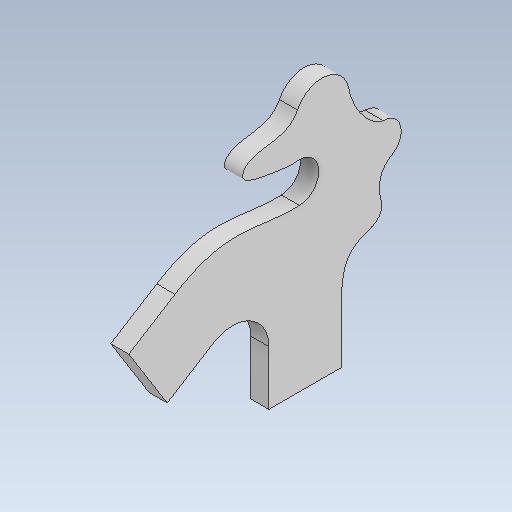
# Autodesk Inventor part: lamina_trasero
Saved by Autodesk Inventor 2021 (Build 250183000, 183)
## iProperties
Created: 2021-04-09
Part Number: lamina_trasero
Material: Genérico
Document SubType Name: Modeling
Designer: j2seb
Density: 1 g/cm^3
Appearance: Valor por defecto
Author: j2seb
Autodesk Inventor part; units mm, degrees
ref_plane "YZ Plane" through (0, 0, 0) normal (1, 0, 0) x (0, 1, 0)
ref_plane "XZ Plane" through (0, 0, 0) normal (0, 1, 0) x (-1, 0, 0)
ref_plane "XY Plane" through (0, 0, 0) normal (0, 0, 1) x (1, 0, 0)
sketch "Boceto1" plane through (0, 0, 0) normal (1, 0, 0) x (0, 1, 0)
  line L0 (525, 5.254) -> (525, 25.254)
  line L1 (525, 25.254) -> (540, 25.254)
  arc A0 (540, 25.254) -> (548.4852, 40.5618) centre (540, 35.2596) ccw
  line L2 (548.4852, 40.5618) -> (540.5364, 53.2825)
  line L3 (540.5364, 53.2825) -> (557.4974, 63.8809)
  line L4 (557.4974, 63.8809) -> (565.4462, 51.1602)
  line L5 (525, 15.254) -> (575, 17.0001) construction
  line L6 (549.0169, 58.5817) -> (575, 17.0001) construction
  line L7 (525, 5.254) -> (540, 5.254)
  circle A1 centre (575, 17.0001) radius 5.5
  line L8 (565.4462, 51.1602) -> (571.7687, 41.0421) construction
  line L9 (569.1709, 26.3286) -> (569.5034, 16.8081) construction
  spline S0 degree 4 poles (565.4462, 51.1602) (571.7687, 41.0421) (572.3019, 33) (569.1709, 26.3286) (569.5034, 16.8081) knots 1 1 1 1 1 2 2 2 2 2
  line L10 (580.3797, 18.1518) -> (580.12, 19.0089) construction
  line L11 (580.12, 19.0089) -> (581.7415, 30.4088) construction
  line L12 (581.7415, 30.4088) -> (583, 33.7094) construction
  line L13 (583, 33.7094) -> (588.2679, 31.7007) construction
  line L14 (588.2679, 31.7007) -> (588, 24.7089) construction
  line L15 (588, 24.7089) -> (589.3884, 18.8714) construction
  line L16 (545.515, 5.254) -> (540, 5.254) construction
  line L17 (571.7687, 41.0421) -> (572.3019, 33) construction
  line L18 (572.3019, 33) -> (569.1709, 26.3286) construction
  arc A2 (590.7303, 3.2162) -> (592.5678, 17.3517) centre (589.3333, 10.585) ccw
  arc A3 (568.8646, -8.7498) -> (578.2128, -6.2962) centre (573.2128, -6.2813) ccw
  arc A4 (554.3846, -3.118) -> (559.2353, -5.7559) centre (558.1928, -1.8941) ccw
  spline S1 degree 4 poles (580.3797, 18.1518) (580.12, 19.0089) (581.7415, 30.4088) (583, 33.7094) (588.2679, 31.7007) (588, 24.7089) (589.3884, 18.8714) (592.5678, 17.3517) knots 0 0 0 0 0 1 2 3 4 4 4 4 4
  line L19 (589.3884, 18.8714) -> (592.5678, 17.3517) construction
  spline S2 degree 4 poles (554.3846, -3.118) (552.5025, 2.7386) (550.3005, 4.7218) (545.515, 5.254) (540, 5.254) knots 21.570729 21.570729 21.570729 21.570729 21.570729 22 22 22 22 22
  line L20 (554.3846, -3.118) -> (552.5025, 2.7386) construction
  line L21 (552.5025, 2.7386) -> (550.3005, 4.7218) construction
  line L22 (550.3005, 4.7218) -> (545.515, 5.254) construction
  line L23 (568.8646, -8.7498) -> (566.1112, -3.8997) construction
  line L24 (566.1112, -3.8997) -> (559.2353, -5.7559) construction
  spline S3 degree 2 poles (568.8646, -8.7498) (566.1112, -3.8997) (559.2353, -5.7559) knots 1 1 1 2 2 2
  line L25 (575, 17.0001) -> (525, 17.0001) construction
  line L26 (590.7303, 3.2162) -> (583.3288, 1.8131) construction
  line L27 (583.3288, 1.8131) -> (578.2201, -3.8262) construction
  line L28 (578.2201, -3.8262) -> (578.2128, -6.2962) construction
  spline S4 degree 3 poles (590.7303, 3.2162) (583.3288, 1.8131) (578.2201, -3.8262) (578.2128, -6.2962) knots 1 1 1 1 2 2 2 2
  point P0 (0, 0)
  point P1 (580.3691, 18.1927)
  point P2 (571.0023, 16.8632)
  dimension "d0" = 20
  dimension "d1" = 60
  dimension "d2" = 15
  dimension "d3" = 11
  dimension "d4" = 15
  dimension "d5" = 10
  dimension "d6" = 8
  dimension "d7" = 2
  dimension "d8" = 50
  constraints: 18 end point, 10 point on circle, 5 centre point, 4 coincident, 4 equal length, 3 horizontal, 3 point on line, 2 midpoint, 2 parallel, 2 perpendicular, 2 tangent, 1 vertical, 25 other
  measures "d0" distance of L7.start L0.end
  measures "d1" angle of L5 L6
  measures "d2" distance of L7.start L16.end
  measures "d3" diameter of A1
  measures "d4" diameter of A2
  measures "d5" diameter of A3
  measures "d6" diameter of A4
  measures "d7" angle of L5 L25
  measures "d8" distance from line of L0 point (575, 17)
extrude "Extrusión1" add sketch "Boceto1" along normal mid plane 5 contours L0 L1 A0 L2 L3 L4 S0 A1 S1 A2 S4 A3 S3 A4 S2 L7
